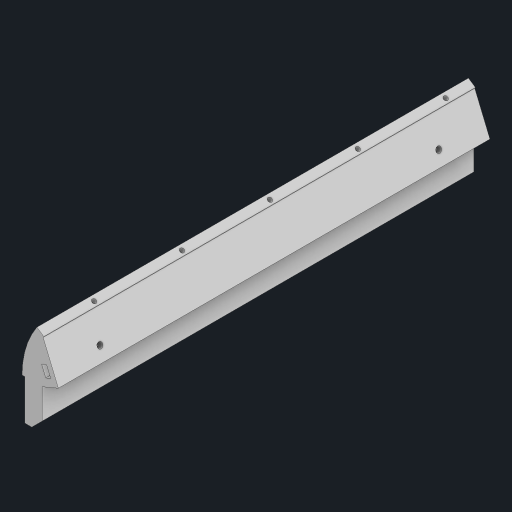
# Autodesk Inventor part: ESQUINA_REDONDEADA_R50_P2
Saved by Autodesk Inventor 2024.3 (Build 283343000, 343)
## iProperties
Created: 2024-05-19
Part Number: ESQUINA_REDONDEADA_R50_P2
Material: Generic
Document SubType Name: Modeling
Designer: Niler
Density: 1 g/cm^3
Appearance: Default
Author: Niler
Autodesk Inventor part; units mm, degrees
ref_plane "YZ Plane" through (0, 0, 0) normal (1, 0, 0) x (0, 1, 0)
ref_plane "XZ Plane" through (0, 0, 0) normal (0, 1, 0) x (-1, 0, 0)
ref_plane "XY Plane" through (0, 0, 0) normal (0, 0, 1) x (1, 0, 0)
ref_plane "Work Plane1" through (0, 0, 0) normal (0, 0, 1) x (1, 0, 0)
sketch "Sketch1" plane through (0, 0, 0) normal (0, 0, 1) x (1, 0, 0)
  line L0 (10, 0) -> (-1.5, 0) projected
  line L1 (10, 45.2667) -> (10, 0) projected
  arc A0 (13.0769, 49.8821) -> (10, 45.2667) centre (15, 45.2667) ccw projected
  line L2 (54.8615, 67.2923) -> (13.0769, 49.8821) projected
  line L3 (50.4385, 77.9077) -> (54.8615, 67.2923) projected
  line L4 (50.4385, 77.9077) -> (29.2692, 69.0872) projected
  arc A1 (29.2692, 69.0872) -> (-1.5, 22.9333) centre (48.5, 22.9333) ccw projected
  line L5 (-1.5, 0) -> (-1.5, 22.9333) projected
  line L6 (15, 45.2667) -> (6.8975, 50.6683)
  line L7 (10, 48.6) -> (19.7692, 25.1538) projected
  line L8 (35.4, 31.6667) -> (10, 21.0833) projected
  line L9 (19.1124, 26.7302) -> (10, 22.9333)
  line L10 (-1.5, 22.9333) -> (10, 22.9333)
  line L11 (-1.5, 22.9333) -> (0, 22.9333)
  line L12 (0, 22.9333) -> (0, -23.4445)
  line L13 (0, -23.4445) -> (-1.5, -23.4445)
  line L14 (-1.5, -23.4445) -> (-1.5, 22.9333)
  line L15 (0, 0.0333) -> (4, 0.0333)
  line L16 (4, 0.0333) -> (10, 6.0333)
  point P0 (0, 0)
  point P1 (10.4897, 47.4247)
  point P2 (10.8397, 48.0402)
  point P3 (10, 48.6)
  point P4 (0, 22.9333)
  dimension "d3" = 1.5
  dimension "d4" = 4
  dimension "d5" = 45
  dimension "d6" = 22.9
  constraints: 18 end point, 4 point on line, 3 parallel, 2 horizontal, 2 perpendicular, 1 point on circle
  measures "d3" distance of L12.end L13.end
  measures "d4" distance of L15.start L15.end
  measures "d5" angle of L1 L16
  measures "d6" distance between parallel lines of L10 L15
extrude "Extrusion1" add sketch "Sketch1" along normal blind 245.5 contours L16 L15 L12 L10 L1 | A1 L6 L7 A0 L1 L10 | L1 A0 L7 L9 | L6 A0 L7
sketch "Sketch2" plane through (6.8975, 50.6683, 245.5) normal (0.5547002, 0.8320503, 0) x (0.8320503, -0.5547002, 0)
  line L0 (4.738, 245.5) -> (0, 245.5) projected
  line L1 (0, 245.5) -> (0, 0) projected
  line L2 (4.738, 0) -> (0, 0) projected
  line L3 (4.738, 245.5) -> (4.738, 0) projected
  circle A0 centre (2.5, 230.5) radius 1.25
  circle A1 centre (2.5, 180.5) radius 1.25
  circle A2 centre (2.5, 130.5) radius 1.25
  circle A3 centre (2.5, 80.5) radius 1.25
  circle A4 centre (2.5, 30.5) radius 1.25
  point P0 (22.3667, 245.5)
  dimension "d7" = 2.5
  dimension "d8" = 2.5
  dimension "d9" = 15
  dimension "d12" = 50
  constraints: 5 centre point, 1 vertical, 8 other
  measures "d7" diameter of A0
  measures "d8" distance from line of L1 A0.centre
  measures "d9" distance from line of L0 A0.centre
  measures "d12" distance of A0.centre A1.centre
extrude "Extrusion2" cut sketch "Sketch2" against normal blind 3 contours A0 | A1 | A2 | A3 | A4
sketch "Sketch3" plane through (0, 0, 0) normal (0, 0, -1) x (-1, 0, 0)
  line L0 (-10, 6.0333) -> (-10, 22.9333) projected
  line L1 (-4, 0.0333) -> (-10, 6.0333) projected
  line L2 (0, 0.0333) -> (-4, 0.0333) projected
  line L3 (0, 22.9333) -> (0, 0.0333) projected
  line L4 (1.5, 22.9333) -> (0, 22.9333) projected
  arc A0 (1.5, 22.9333) -> (-6.8975, 50.6683) centre (-48.5, 22.9333) ccw projected
  line L5 (-10.8397, 48.0402) -> (-6.8975, 50.6683) projected
  arc A1 (-10.4897, 47.4247) -> (-10.8397, 48.0402) centre (-15, 45.2667) ccw projected
  line L6 (-19.1124, 26.7302) -> (-10.4897, 47.4247) projected
  line L7 (-10, 22.9333) -> (-19.1124, 26.7302) projected
  line L8 (-12.4384, 34.9479) -> (-14.7461, 29.4095)
  line L9 (-14.7461, 29.4095) -> (-11.9768, 28.2556)
  line L10 (-11.9768, 28.2556) -> (-9.6691, 33.7941)
  line L11 (-9.6691, 33.7941) -> (-12.4384, 34.9479)
  point P0 (0, 0)
  dimension "d19" = 12.7
  dimension "d20" = 6
  dimension "d21" = 3
  dimension "d22" = 3
  constraints: 8 end point, 3 perpendicular, 1 parallel
  measures "d19" distance from line of L5.start L11
  measures "d20" distance of L9.end L10.end
  measures "d21" distance of L8.end L9.end
  measures "d22" distance between parallel lines of L6 L8
extrude "Extrusion3" cut sketch "Sketch3" against normal blind 30 contours L11 L10 L9 L8
sketch "Sketch4" plane through (10.4897, 47.4247, 245.5) normal (0.9230769, 0.3846154, 0) x (0, 0, -1)
  line L0 (245.5, -22.4191) -> (245.5, 0) projected
  line L1 (245.5, 0) -> (0, 0) projected
  line L2 (0, -22.4191) -> (0, 0) projected
  line L3 (245.5, -22.4191) -> (0, -22.4191) projected
  line L4 (245.5, -18.2665) -> (245.5, -12.2665) construction
  line L5 (245.5, -18.2665) -> (215.5, -18.2665) projected
  line L6 (215.5, -18.2665) -> (215.5, -12.2665) projected
  line L7 (245.5, -12.2665) -> (215.5, -12.2665) projected
  circle A0 centre (219.1, -15.2665) radius 1.65
  line L8 (220.7743, -18.1665) -> (217.4257, -18.1665)
  line L9 (217.4257, -18.1665) -> (215.7514, -15.2665)
  line L10 (215.7514, -15.2665) -> (217.4257, -12.3665)
  line L11 (217.4257, -12.3665) -> (220.7743, -12.3665)
  line L12 (220.7743, -12.3665) -> (222.4486, -15.2665)
  line L13 (222.4486, -15.2665) -> (220.7743, -18.1665)
  point P0 (245.5, -39.7422)
  point P1 (215.5, -15.2665)
  dimension "d25" = 3.3
  dimension "d26" = 3.6
  dimension "d27" = 5.8
  constraints: 12 end point, 2 horizontal alignment, 1 centre point, 1 coincident, 1 midpoint, 13 other
  measures "d25" diameter of A0
  measures "d26" distance from line of L6 A0.centre
  measures "d27" distance between parallel lines of L11 L8
extrude "Extrusion4" cut sketch "Sketch4" against normal blind 7 contours A0
ref_plane "Work Plane2" through (0, 0, 122.75) normal (0, 0, 1) x (1, 0, 0)
mirror "Mirror1" about plane through (0, 0, 122.75) normal (0, 0, 1) of "Extrusion4", "Extrusion3"
body "Solid1"
